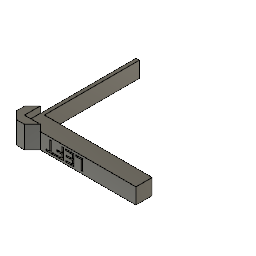
Alignment guide (Autodesk Fusion 360 design; units mm, degrees)
Autodesk Fusion 360 part; units mm, degrees
sketch "Schizzo1" plane through (0, 0, 0) normal (0, 0, 1) x (1, 0, 0)
  line L0 (0, 0) -> (40, 0)
  line L1 (40, 0) -> (40, 7.3)
  line L2 (40, 7.3) -> (0, 7.3)
  line L3 (0, 7.3) -> (0, 0)
  line L4 (0, 0) -> (2.2, 0)
  line L5 (2.2, 0) -> (2.2, 40)
  line L6 (2.2, 40) -> (0, 40)
  line L7 (0, 40) -> (0, 0)
  line L8 (0, 17.3) -> (0, 7.3)
  line L9 (0, 0) -> (10, 0)
  line L10 (10, 0) -> (10, -5)
  line L11 (10, -5) -> (0, -5)
  line L12 (0, -5) -> (0, 0)
  line L13 (0, -5) -> (-5, -5)
  line L14 (-5, -5) -> (-5, 10.2705)
  line L15 (-5, 10.2705) -> (0, 10.2705)
  line L16 (0, 10.2705) -> (0, -5)
  dimension "d1" = 40
  dimension "d2" = 7.3
  dimension "d3" = 2.2
  dimension "d4" = 40
  dimension "d6" = 10
  dimension "d7" = 10
  dimension "d8" = 5
  dimension "d9" = 5
  constraint horizontal L0
  constraint vertical L1
  constraint horizontal L2
  constraint vertical L3
  constraint coincident L0.start L3.end
  constraint horizontal L4
  constraint vertical L5
  constraint horizontal L6
  constraint vertical L7
  constraint vertical L8
  constraint horizontal L9
  constraint vertical L10
  constraint horizontal L11
  constraint vertical L12
  constraint horizontal L13
  constraint vertical L14
  constraint horizontal L15
  constraint vertical L16
  measures "d1" distance of L0.start L0.end
  measures "d2" distance of L0.start L2.end
  measures "d3" distance of L0.start L4.end
  measures "d4" distance of L0.start L6.end
  measures "d6" distance of L2.end L8.start
  measures "d7" distance of L0.start L9.end
  measures "d8" distance of L0.start L11.end
  measures "d9" distance of L11.end L13.end
extrude "Estrusione1" add sketch "Schizzo1" along normal blind 10
extrude "Estrusione2" add sketch "Schizzo1" along normal blind 14 contours L3 L7 L8 L12 L13 L14 L15 L16 | L0 L4 L9 L10 L11 L12 L16
chamfer "Smusso1" distance 5 angle 45 2 edges at (-5, 10.2705, 7) (10, -5, 7)
chamfer "Smusso2" distance 5 angle 45 1 edges at (-5, -5, 7)
sketch "Schizzo2" plane through (0, 0, 0) normal (0, -1, 0) x (1, 0, 0)
  line L0 (10, 0) -> (40, 0)
  line L1 (40, 0) -> (40, 10)
  line L2 (40, 10) -> (10, 10)
  line L3 (10, 10) -> (10, 0)
  line L4 (40, 10.0237) -> (10, 10.0237) construction
  line L5 (10, 10.0237) -> (10, 0) construction
  line L6 (10, 0) -> (40, 0) construction
  line L7 (40, 0) -> (40, 10.0237) construction
  dimension "d16" = 7
  text T0 "LEFT" font "Arial" height 7 align centre middle in box 30 x 10.0237 at (40, 10.0237) x (-1, 0) y (0, -1) spacing 1
  constraint coincident L0.end
  constraint midpoint L0
extrude "Estrusione3" cut sketch "Schizzo2" against normal blind 3 text T0
move_face "FacceDiOffset1" offset 3 1 faces at (27.4, 7.3, 3.3333)
move_face "FacceDiOffset2" offset 30 1 faces at (40, 3.4333, 3.3333)
move_face "FacceDiOffset3" offset 30 1 faces at (1.4667, 40, 6.6667)
